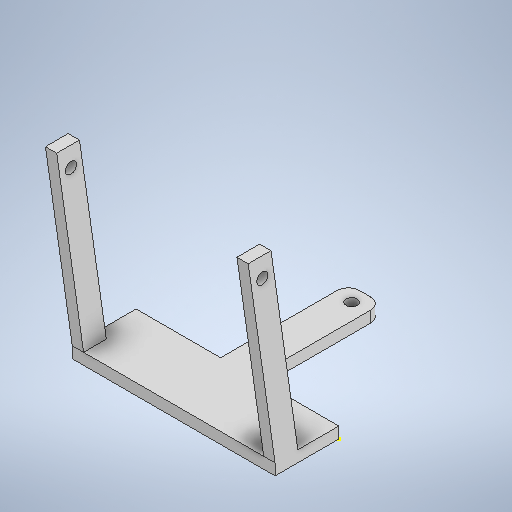
# Autodesk Inventor part: SERVO CUELLO
Saved by Autodesk Inventor 2025.3 (Build 293356030, 356C)
## iProperties
Created: 2026-07-17
Part Number: SERVO CUELLO
Material: Generic
Document SubType Name: Modeling
Designer: Samuel Correa Vega
Density: 1 g/cm^3
Appearance: Default
Author: Samuel Correa Vega
Autodesk Inventor part; units mm, degrees
ref_plane "YZ Plane" through (0, 0, 0) normal (1, 0, 0) x (0, 1, 0)
ref_plane "XY Plane" through (0, 0, 0) normal (0, 0, 1) x (1, 0, 0)
sketch "Sketch1" plane through (0, 0, 0) normal (0, 1, 0) x (-1, 0, 0)
  line L0 (3.0863, 11.3309) -> (-2.9137, 11.3309)
  line L1 (-2.9137, 11.3309) -> (-2.9137, -22.6691)
  line L2 (-2.9137, -22.6691) -> (3.0863, -22.6691)
  line L3 (3.0863, -22.6691) -> (3.0863, 11.3309)
  point P0 (0, 0)
  dimension "d0" = 6
  dimension "d1" = 34
  constraints: 8 end point, 2 parallel, 1 horizontal, 1 perpendicular
  measures "d0" distance of L0.start L0.end
  measures "d1" distance of L2.end L0.start
extrude "Extrusion1" add sketch "Sketch1" along normal blind 2
fillet "Fillet1" radius 2 2 edges at (2.9137, 1, -22.6691) (-3.0863, 1, -22.6691)
ref_plane "Work Plane1" through (0, 2, 0) normal (0, 1, 0) x (-1, 0, 0)
sketch "Sketch2" plane through (0, 0, 0) normal (0, 0, 1) x (1, 0, 0)
  line L0 (-3.0863, 0) -> (-3.0863, 2) projected
  line L1 (-16.0863, 2) -> (-16.0863, 35)
  line L2 (-16.0863, 35) -> (-18.0863, 35)
  line L3 (-18.0863, 35) -> (-18.0863, 0)
  line L4 (15.9137, 2) -> (15.9137, 35)
  line L5 (15.9137, 35) -> (17.9137, 35)
  line L6 (17.9137, 35) -> (17.9137, 0)
  line L7 (-18.0863, 2.3607) -> (-18.0863, 0)
  line L8 (-18.0863, 0) -> (-3.0863, 0)
  line L9 (-3.0863, 2) -> (-16.0863, 2)
  line L10 (2.9137, 2) -> (15.9137, 2)
  line L11 (17.9137, 2) -> (17.9137, 0)
  line L12 (17.9137, 0) -> (2.9137, 0)
  line L13 (-3.0863, 2) -> (2.9137, 2) projected
  line L14 (2.9137, 2) -> (2.9137, 0)
  point P0 (0, 0)
  point P1 (-17.0863, 35)
  point P2 (16.9137, 35)
  point P3 (-0.0863, 2)
  dimension "d6" = 2
  dimension "d7" = 2
  dimension "d8" = 35
  dimension "d14" = 32
  constraints: 26 end point, 5 point on line, 4 vertical, 3 equal length, 3 horizontal alignment, 3 midpoint, 3 parallel, 2 perpendicular
  measures "d6" distance of L1.end L2.end
  measures "d7" distance of L4.end L5.end
  measures "d8" distance of L3.end L2.end
  measures "d14" distance between parallel lines of L4 L1
extrude "Extrusion2" add sketch "Sketch2" along normal blind 16.0935
sketch "Sketch4" plane through (15.9137, 2, 0) normal (-1, 0, 0) x (0, 0, 1)
  line L0 (16.0935, 33) -> (16.0935, 0) projected
  line L1 (11.3309, 0) -> (16.0935, 33)
  line L2 (16.0935, 33) -> (11.3309, 0)
  line L3 (11.3309, -2) -> (11.3309, 0) projected
  line L4 (0, -2) -> (16.0935, -2) projected
  line L5 (11.3309, -2) -> (16.0935, -2)
  line L6 (16.0935, -2) -> (16.0935, 33)
  constraints: 8 end point, 2 collinear, 1 perpendicular
extrude "Extrusion4" cut sketch "Sketch4" along normal through all both and the other way through all
sketch "Sketch5" plane through (-18.0863, 0, 0) normal (-1, 0, 0) x (0, 0, 1)
  line L0 (0, 2) -> (11.3309, 2) projected
  line L1 (7.2895, 2) -> (12.0521, 35)
  line L2 (0, 35) -> (16.0935, 35) projected
  line L3 (7.2895, 2) -> (0, 2)
  line L4 (0, 2) -> (0, 35)
  line L5 (0, 35) -> (12.0521, 35)
  line L6 (11.3309, 2) -> (16.0935, 35) projected
  point P0 (0, 0)
  dimension "d17" = 4
  constraints: 8 end point, 2 perpendicular, 2 point on line, 1 horizontal, 1 parallel
  measures "d17" distance between parallel lines of L6 L1
extrude "Extrusion5" cut sketch "Sketch5" along normal through all both and the other way through all contours L4 L2 L1 L0
sketch "Sketch6" plane through (17.9137, 0, 0) normal (1, 0, 0) x (0, 0, -1)
  point P0 (0, 0)
sketch "Sketch7" plane through (0, 2, 0) normal (0, 1, 0) x (1, 0, 0)
  circle A0 centre (0, 5.6924) radius 1
  circle A1 centre (0, 20.1644) radius 1
  line L0 (0.9137, 22.6691) -> (-1.0863, 22.6691) projected
  line L1 (2.9137, 0) -> (2.9137, 20.6691) projected
  point P0 (0, 0)
  point P1 (-0.0863, 22.6691)
  dimension "d20" = 2
  dimension "d21" = 2
  dimension "d24" = 2.5047
  dimension "d25" = 2.9137
  dimension "d26" = 14.472
  constraints: 2 centre point, 1 midpoint
  measures "d20" diameter of A1
  measures "d21" diameter of A0
  measures "d24" vertical distance of point (-0.086, 22.669) A1.centre
  measures "d25" distance from line of L1 A1.centre
  measures "d26" distance of A0.centre A1.centre
extrude "Extrusion6" cut sketch "Sketch7" against normal through all
sketch "Sketch9" plane through (17.9137, 0, 0) normal (1, 0, 0) x (0, 0, -1)
  circle A0 centre (-13.5677, 31.5) radius 1
  line L0 (-12.0521, 35) -> (-16.0935, 35) projected
  line L1 (-14.0728, 35) -> (-9.0138, -0.0536) construction
  line L2 (-16.0935, 35) -> (-11.3309, 2) projected
  point P0 (0, 0)
  dimension "d30" = 2
  dimension "d31" = 3.5
  constraints: 2 end point, 1 centre point, 1 midpoint, 1 parallel, 1 point on line
  measures "d30" diameter of A0
  measures "d31" vertical distance of L1.start A0.centre
extrude "Extrusion8" cut sketch "Sketch9" against normal through all
body "Solid1"
